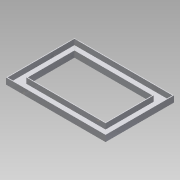
# Autodesk Inventor part: Catch pan
Saved by Autodesk Inventor 2015 (Build 190159000, 159)
## iProperties
Created: 2015-05-27
Part Number: Catch pan
Material: Aluminum 6061
Document SubType Name: Modeling
Designer: Joe Sheldon
Density: 2.7 g/cm^3
Appearance: Aluminum - Flat
Author: Joe Sheldon
Autodesk Inventor part; units mm, degrees
ref_plane "YZ Plane" through (0, 0, 0) normal (1, 0, 0) x (0, 1, 0)
ref_plane "XZ Plane" through (0, 0, 0) normal (0, 1, 0) x (-1, 0, 0)
ref_plane "XY Plane" through (0, 0, 0) normal (0, 0, 1) x (1, 0, 0)
sketch "Sketch3" plane through (0, 0, 0) normal (0, 1, 0) x (-1, 0, 0)
  line L0 (-203.2, 139.7) -> (203.2, 139.7)
  line L1 (203.2, 139.7) -> (203.2, -139.7)
  line L2 (203.2, -139.7) -> (-203.2, -139.7)
  line L3 (-203.2, -139.7) -> (-203.2, 139.7)
  line L4 (-203.2, 139.7) -> (203.2, -139.7) construction
  line L5 (203.2, 139.7) -> (-203.2, -139.7) construction
  line L6 (152.4, -88.9) -> (152.4, 88.9)
  line L7 (152.4, 88.9) -> (-152.4, 88.9)
  line L8 (-152.4, 88.9) -> (-152.4, -88.9)
  line L9 (-152.4, -88.9) -> (152.4, -88.9)
  line L10 (158.75, -95.25) -> (158.75, 95.25)
  line L11 (158.75, 95.25) -> (-158.75, 95.25)
  line L12 (-158.75, 95.25) -> (-158.75, -95.25)
  line L13 (-158.75, -95.25) -> (158.75, -95.25)
  point P0 (0, 0)
  dimension "d11" = 406.4
  dimension "d12" = 279.4
  dimension "d13" = 50.8
  dimension "d14" = 44.45
  constraints: 28 end point, 6 parallel, 3 perpendicular, 2 midpoint, 1 horizontal, 6 other
  measures "d11" distance of L1.end L2.end
  measures "d12" distance of L0.end L1.end
  measures "d13" distance between parallel lines of L1 L6
  measures "d14" distance between parallel lines of L1 L10
extrude "Extrusion3" add sketch "Sketch3" along normal blind 50.8 contours L0 L1 L2 L3
shell "Shell2" thickness 3.175 removed faces 1 at (52.9167, 50.8, -124.8833)
sketch "Sketch4" plane through (0, 50.8, 0) normal (0, 1, 0) x (1, 0, 0)
  line L0 (227.9599, -165.6341) -> (-227.9599, -165.6341)
  line L1 (-227.9599, -165.6341) -> (-227.9599, 165.6341)
  line L2 (-227.9599, 165.6341) -> (227.9599, 165.6341)
  line L3 (227.9599, 165.6341) -> (227.9599, -165.6341)
  line L4 (227.9599, -165.6341) -> (-227.9599, 165.6341) construction
  line L5 (-227.9599, -165.6341) -> (227.9599, 165.6341) construction
  point P0 (0, 0)
  constraints: 12 end point, 2 midpoint, 2 parallel, 1 horizontal, 1 perpendicular
extrude "Extrusion4" cut sketch "Sketch4" against normal blind 25.4
body "Solid3"
